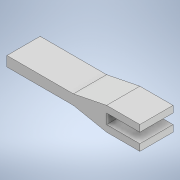
# Autodesk Inventor part: MotorHållare
Saved by Autodesk Inventor 2021 (Build 250183000, 183)
## iProperties
Created: 2025-01-15
Part Number: MotorHållare
Material: Generic
Document SubType Name: Modeling
Designer: 24oscnor
Density: 1 g/cm^3
Appearance: Default
Author: 24oscnor
Autodesk Inventor part; units mm, degrees
ref_plane "YZ Plane" through (0, 0, 0) normal (1, 0, 0) x (0, 1, 0)
ref_plane "XZ Plane" through (0, 0, 0) normal (0, 1, 0) x (-1, 0, 0)
ref_plane "XY Plane" through (0, 0, 0) normal (0, 0, 1) x (1, 0, 0)
sketch "Sketch1" plane through (0, 0, 0) normal (0, 1, 0) x (-1, 0, 0)
  line L0 (0, 0) -> (30, 0)
  line L1 (30, 0) -> (30, 10)
  line L2 (30, 10) -> (0, 10)
  line L3 (0, 10) -> (0, 0)
  dimension "d0" = 30
  dimension "d1" = 10
  constraints: 8 end point, 2 parallel, 1 horizontal, 1 perpendicular
  measures "d0" distance of L1.end L2.end
  measures "d1" distance of L2.end L0.start
extrude "Extrusion1" add sketch "Sketch1" along normal blind 3
sketch "Sketch2" plane through (0, 3, 0) normal (0, 1, 0) x (1, 0, 0)
  line L0 (-30, -10) -> (0, -10) projected
  line L1 (-10, -10) -> (10, -10)
  line L2 (10, -10) -> (10, 0)
  line L3 (10, 0) -> (-10, 0)
  line L4 (-10, 0) -> (-10, -10)
  line L5 (0, -10) -> (0, 0) projected
  dimension "d4" = 10
  dimension "d5" = 10
  dimension "d6" = 20
  constraints: 8 end point, 2 parallel, 1 horizontal, 1 perpendicular, 1 point on line
  measures "d4" distance between parallel lines of L4 L5
  measures "d5" distance between parallel lines of L5 L2
  measures "d6" distance of L2.end L3.end
extrude "Extrusion2" add sketch "Sketch2" along normal blind 2
sketch "Sketch3" plane through (0, 0, 0) normal (0, -1, 0) x (1, 0, 0)
  line L0 (-10, 10) -> (10, 10) projected
  line L1 (10, 0) -> (0, 0) projected
  line L2 (-10, 10) -> (10, 10)
  line L3 (10, 10) -> (10, 0)
  line L4 (10, 0) -> (-10, 0)
  line L5 (-10, 0) -> (-10, 10)
  constraints: 8 end point, 2 parallel, 1 horizontal, 1 perpendicular
extrude "Extrusion3" add sketch "Sketch3" along normal blind 2
sketch "Sketch4" plane through (-30, 0, 10) normal (0, 0, 1) x (1, 0, 0)
  line L0 (20, 0) -> (20, -2) projected
  line L1 (20, 0) -> (30, -2)
  line L2 (40, -2) -> (20, -2) projected
  line L3 (0, 3) -> (20, 3) projected
  line L4 (20, 3) -> (30, 5)
  line L5 (20, 5) -> (40, 5) projected
  line L6 (30, 3) -> (30, 5)
  line L7 (30, 3) -> (20, 3)
  line L8 (30, 0) -> (30, 3) projected
  line L9 (30, -2) -> (30, 0)
  line L10 (30, 0) -> (20, 0)
  line L11 (20, 3) -> (20, 5) projected
  line L12 (20, 3) -> (20, 5)
  line L13 (20, 5) -> (30, 5)
  line L14 (30, -2) -> (20, -2)
  line L15 (20, -2) -> (20, 0)
  constraints: 20 end point, 4 perpendicular, 2 midpoint, 2 vertical, 1 collinear
extrude "Extrusion4" cut sketch "Sketch4" against normal through all contours L1 L2 L0 | L4 L11 L5
body "Solid1"
